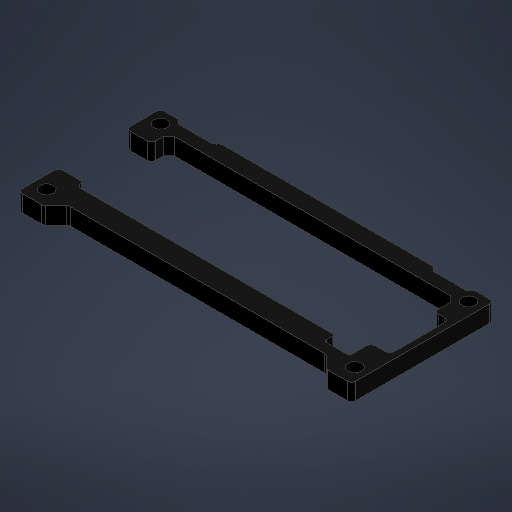
# Autodesk Inventor part: DribblerVerbindungV2
Saved by Autodesk Inventor 2025.2 (Build 292293000, 293)
## iProperties
Created: 2024-12-09
Part Number: DribblerVerbindungV2
Material: Generisch
Document SubType Name: Modeling
Designer: Fabian
Density: 1 g/cm^3
Appearance: Vorgabe
Author: Fabian
Autodesk Inventor part; units mm, degrees
ref_plane "YZ Plane" through (0, 0, 0) normal (1, 0, 0) x (0, 1, 0)
ref_plane "XZ Plane" through (0, 0, 0) normal (0, 1, 0) x (-1, 0, 0)
ref_plane "XY Plane" through (0, 0, 0) normal (0, 0, 1) x (1, 0, 0)
sketch "Skizze1" plane through (0, 0, 0) normal (0, 1, 0) x (-1, 0, 0)
  line L0 (-33.55, 10.5) -> (-33.55, 3.838)
  line L1 (33.55, 4.938) -> (33.55, 10.5)
  line L2 (-39.55, 16.5) -> (-39.55, -16.5)
  line L3 (-39.55, -16.5) -> (39.55, -16.5)
  line L4 (39.55, -16.5) -> (39.55, 16.5)
  line L5 (-39.55, 17.265) -> (39.55, 17.265)
  line L6 (39.55, 17.265) -> (39.55, 16.5)
  line L7 (-39.55, 17.265) -> (-39.55, 16.5)
  line L8 (-38.05, -3.162) -> (-38.05, -10.162)
  line L9 (-38.05, -3.162) -> (-38.05, 3.838)
  line L10 (-38.05, 3.838) -> (-36.55, 3.838)
  line L11 (-36.55, 3.838) -> (-33.55, 3.838)
  line L12 (-38.05, -10.162) -> (-34.55, -10.162)
  line L13 (-34.55, -10.162) -> (-34.55, -11.262)
  line L14 (37.5501, -3.145) -> (37.5501, -11.262)
  line L15 (37.5501, -3.145) -> (37.5501, 4.938)
  line L16 (37.5501, 4.938) -> (33.55, 4.938)
  line L17 (0, 13.265) -> (33.55, 13.265)
  line L18 (33.55, 13.265) -> (33.55, 10.5)
  line L19 (0, 13.265) -> (-33.55, 13.265)
  line L20 (-33.55, 13.265) -> (-33.55, 10.5)
  line L21 (33.55, -13.5) -> (33.55, -16.5)
  line L22 (33.55, -16.5) -> (33.55, -12.5)
  line L23 (33.55, -12.5) -> (33.55, -11.262)
  line L24 (33.55, -12.5) -> (-34.55, -12.5)
  line L25 (-34.55, -12.5) -> (-34.55, -11.262)
  line L26 (37.5501, -11.262) -> (33.55, -11.262)
  line L27 (-39.55, -16.5) -> (-34.55, -16.5)
  line L28 (-39.55, -16.5) -> (-34.55, -16.5)
  line L29 (-34.55, -16.5) -> (-34.55, -13.5)
  line L30 (-34.55, -13.5) -> (-25.55, -13.5)
  line L31 (-25.55, -13.5) -> (-25.55, -16.5)
  line L32 (39.55, -16.5) -> (34.55, -16.5)
  line L33 (34.55, -16.5) -> (34.55, -13.5)
  line L34 (34.55, -13.5) -> (25.55, -13.5)
  line L35 (25.55, -13.5) -> (25.55, -16.5)
  line L36 (-25.55, -16.5) -> (-25.55, -15.5)
  line L37 (-25.55, -15.5) -> (-34.55, -15.5)
  line L38 (25.55, -16.5) -> (25.55, -15.5)
  line L39 (25.55, -15.5) -> (34.55, -15.5)
  line L40 (-36.55, 13.5) -> (-36.55, -0.332)
  line L41 (-36.55, -0.332) -> (-36.55, 6.668)
  line L42 (-36.55, -0.332) -> (-36.55, -7.332)
  line L43 (-34.55, -10.162) -> (-34.55, -7.332)
  line L44 (-34.55, -7.332) -> (-38.05, -7.332)
  line L45 (-36.55, 6.668) -> (-38.05, 6.668)
  line L46 (-38.05, 6.668) -> (-38.05, 3.838)
  line L47 (-36.55, 6.668) -> (-33.55, 6.668)
  line L48 (36.55, 13.5) -> (36.55, -0.332)
  line L49 (36.55, -0.332) -> (36.55, 7.668)
  line L50 (36.55, -0.332) -> (36.55, -8.332)
  line L51 (36.55, -8.332) -> (33.55, -8.332)
  line L52 (33.55, -8.332) -> (33.55, -11.262)
  line L53 (36.55, -8.332) -> (37.5501, -8.332)
  line L54 (36.55, 7.668) -> (33.55, 7.719)
  line L55 (37.5501, 4.938) -> (37.5501, 7.668)
  line L56 (37.5501, 7.668) -> (36.55, 7.668)
  line L57 (37.5501, -8.332) -> (39.55, -8.332)
  line L58 (37.5501, 7.668) -> (39.55, 7.668)
  line L59 (0, 13.265) -> (0, 9.265)
  line L60 (33.55, 9.265) -> (-33.55, 9.265)
  line L61 (33.55, 13.265) -> (33.55, 14.265)
  line L62 (33.55, 14.265) -> (-33.55, 14.265)
  line L63 (-33.55, 14.265) -> (-33.55, 13.265)
  line L64 (33.55, 17.265) -> (30.55, 14.265)
  line L65 (33.55, 17.265) -> (37.7926, 17.265) construction
  line L66 (-33.55, 17.265) -> (-30.55, 14.265)
  point P0 (0, 0)
  point P1 (36.55, -13.5)
  point P2 (-36.55, -13.5)
  dimension "d28" = 3
  dimension "d29" = 4
  dimension "d32" = 5
  dimension "d33" = 3
  dimension "d34" = 9
  dimension "d35" = 5
  dimension "d36" = 3
  dimension "d37" = 9
  dimension "d45" = 1
  dimension "d46" = 1
  dimension "d47" = 13.832
  dimension "d48" = 7
  dimension "d49" = 7
  dimension "d50" = 13.832
  dimension "d51" = 8
  dimension "d52" = 8
  dimension "d55" = 4
  dimension "d56" = 1
  dimension "d58" = 135
  constraints: 134 end point, 24 perpendicular, 24 point on line, 10 vertical, 5 horizontal, 5 parallel, 2 symmetric about line, 1 collinear, 1 equal length, 1 midpoint
  measures "d28" distance of point (36.55, -13.5) L21.start
  measures "d29" distance of L21.end L22.end
  measures "d32" distance of L2.end L27.end
  measures "d33" distance of L27.end L29.end
  measures "d34" distance of L29.end L30.end
  measures "d35" distance of L3.end L32.end
  measures "d36" distance of L32.end L33.end
  measures "d37" distance of L33.end L34.end
  measures "d45" distance of L31.end L36.end
  measures "d46" distance of L35.end L38.end
  measures "d47" distance of L40.start L40.end
  measures "d48" distance of L40.end L41.end
  measures "d49" distance of L40.end L42.end
  measures "d50" distance of L48.start L48.end
  measures "d51" distance of L48.end L49.end
  measures "d52" distance of L48.end L50.end
  measures "d55" distance of L17.start L59.end
  measures "d56" distance of L17.end L61.end
  measures "d58" angle of L64 L65
extrude "Extrusion1" add sketch "Skizze1" against normal blind 4 contours L20 L19 L59 L60 L0 | L0 L47 L45 L46 L9 L8 L12 L13 L25 L24 L22 L34 L35 L3 L31 L30 L29 L2 L7 L5 L66 L62 L63 L20 | L63 L62 L61 L17 L19 | L59 L17 L18 L1 L60 | L1 L18 L61 L62 L64 L5 L6 L4 L58 L56 L54 | L44 L43 L12 L8 | L53 L14 L26 L52 L51 | L4 L3 L33 L34 L22 L23 L26 L14 L57 | L29 L30 L31 L37 | L39 L21 L34 L33 | L35 L34 L21 L39
hole "Bohrung1" at (-36.55, 0, -13.5) at (36.55, 0, -13.5) at (36.55, 0, 13.5) at (-36.55, 0, 13.5) direction (0, -1, 0) diameter 3.2 depth 6 tip angle 118
chamfer "Fasen1" distance 1.238 angle 45 2 edges at (-33.55, -2, -12.5) (34.55, -2, -12.5)
chamfer "Fasen2" distance 0.5 angle 45 1 edges at (-33.55, -2, 9.265)
fillet "Rundung1" radius 1 16 edges at (39.55, -2, 17.265) (39.55, -2, -16.5) (-39.55, -2, 17.265) (-39.55, -2, -16.5) (-34.55, -2, -16.5) (-25.55, -2, -16.5) (25.55, -2, -16.5) (34.55, -2, -16.5) (25.55, -2, -15.5) (34.55, -2, -15.5) (-34.55, -2, -15.5) (-25.55, -2, -15.5) (-33.55, -2, 17.265) (-30.55, -2, 14.265) (33.55, -2, 17.265) (30.55, -2, 14.265)
fillet "Rundung2" radius 1 8 edges at (-33.55, -2, -8.332) (-33.55, -2, 7.719) (33.55, -2, 6.668) (34.55, -2, -7.332) (38.05, -2, -7.332) (38.05, -2, 6.668) (-39.55, -2, 7.668) (-39.55, -2, -8.332)
sketch "Skizze3" plane through (0, -4, 0) normal (0, -1, 0) x (1, 0, 0)
  line L0 (33.55, 7.668) -> (33.55, 9.265) projected
  line L1 (33.55, 9.265) -> (27.55, 9.265)
  line L2 (27.55, 9.265) -> (27.55, 11.765)
  line L3 (27.55, 11.765) -> (33.55, 11.765)
  line L4 (33.55, 11.765) -> (33.55, 9.265)
  point P0 (0, 0)
  dimension "d59" = 6
  dimension "d60" = 2.5
  constraints: 8 end point, 2 parallel, 1 horizontal, 1 perpendicular
  measures "d59" distance of L2.end L3.end
  measures "d60" distance of L1.end L2.end
extrude "Extrusion2" cut sketch "Skizze3" against normal blind 4
fillet "Rundung3" radius 0.5 3 edges at (33.55, -2, 11.765) (27.55, -2, 11.765) (27.55, -2, 9.265)
